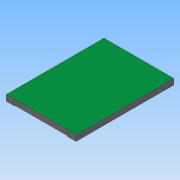
# Autodesk Inventor part: NINA-W102 Body
Saved by Autodesk Inventor 2016 (Build 200138000, 138)
## iProperties
Created: 2019-08-17
Part Number: NINA-W102 Body
Material: Generic
Document SubType Name: Modeling
Designer: Orest
Mass: 0.113046 g
Surface Area: 3.2498 cm^2
Volume: 0.113046 cm^3
Density: 1 g/cm^3
Appearance: Default
Author: Orest
Autodesk Inventor part; units mm, degrees
ref_plane "YZ Plane" through (0, 0, 0) normal (1, 0, 0) x (0, 1, 0)
ref_plane "XZ Plane" through (0, 0, 0) normal (0, 1, 0) x (-1, 0, 0)
ref_plane "XY Plane" through (0, 0, 0) normal (0, 0, 1) x (1, 0, 0)
sketch "Sketch10" plane through (0, 0, 0) normal (0, 1, 0) x (-1, 0, 0)
  line L0 (7, -5) -> (-7, -5)
  line L1 (-7, -5) -> (-7, 5)
  line L2 (-7, 5) -> (7, 5)
  line L3 (6.9, -3.35) -> (6.9, 3.35)
  line L4 (7, 5) -> (7, 3.9745)
  line L5 (7, -3.9745) -> (7, -5)
  line L6 (-7, 0) -> (6.9, 0) construction
  arc A0 (6.9, -3.35) -> (7, -3.9745) centre (8.9, -3.35) ccw
  arc A1 (7, 3.9745) -> (6.9, 3.35) centre (8.9, 3.35) ccw
  point P0 (0, 0)
  point P1 (0, -5)
  dimension "d7" = 14
  dimension "d8" = 10
  dimension "d9" = 0.1
  dimension "d11" = 1.65
  dimension "d12" = 2
  constraints: 14 end point, 4 point on circle, 3 midpoint, 3 parallel, 2 centre point, 2 horizontal, 1 collinear, 1 horizontal alignment, 1 perpendicular, 1 tangent, 1 vertical, 1 vertical alignment, 1 other
  measures "d7" distance of L1.end L2.end
  measures "d8" distance of L0.end L1.end
  measures "d9" distance between parallel lines of L3 L4
  measures "d11" distance from line of L3.start L0
  measures "d12" radius of A0
extrude "Extrusion4" add sketch "Sketch10" along normal blind 0.8
sketch "Sketch11" plane through (0, 0, 0) normal (0, -1, 0) x (1, 0, 0)
  line L0 (-6.45, 4.7) -> (-5.75, 4.7)
  line L1 (-5.75, 4.7) -> (-5.75, 3.55)
  line L2 (-5.75, 3.55) -> (-6.45, 3.55)
  line L3 (-6.45, 3.55) -> (-6.45, 4.7)
  line L4 (-7, -5) -> (7, -5) construction
  line L5 (7, -5) -> (7, 5) construction
  line L6 (7, 5) -> (-7, 5) construction
  line L7 (-7, 5) -> (-7, 3.9745) construction
  arc A0 (-6.9, 3.35) -> (-7, 3.9745) centre (-8.9, 3.35) ccw construction
  line L8 (-6.9, 3.35) -> (-6.9, -3.35) construction
  arc A1 (-7, -3.9745) -> (-6.9, -3.35) centre (-8.9, -3.35) ccw construction
  line L9 (-7, -3.9745) -> (-7, -5) construction
  line L10 (-5.45, 4.7) -> (-4.75, 4.7)
  line L11 (-4.75, 4.7) -> (-4.75, 3.55)
  line L12 (-4.75, 3.55) -> (-5.45, 3.55)
  line L13 (-5.45, 3.55) -> (-5.45, 4.7)
  line L14 (-4.45, 4.7) -> (-3.75, 4.7)
  line L15 (-3.75, 4.7) -> (-3.75, 3.55)
  line L16 (-3.75, 3.55) -> (-4.45, 3.55)
  line L17 (-4.45, 3.55) -> (-4.45, 4.7)
  line L18 (-3.45, 4.7) -> (-2.75, 4.7)
  line L19 (-2.75, 4.7) -> (-2.75, 3.55)
  line L20 (-2.75, 3.55) -> (-3.45, 3.55)
  line L21 (-3.45, 3.55) -> (-3.45, 4.7)
  line L22 (-2.45, 4.7) -> (-1.75, 4.7)
  line L23 (-1.75, 4.7) -> (-1.75, 3.55)
  line L24 (-1.75, 3.55) -> (-2.45, 3.55)
  line L25 (-2.45, 3.55) -> (-2.45, 4.7)
  line L26 (-1.45, 4.7) -> (-0.75, 4.7)
  line L27 (-0.75, 4.7) -> (-0.75, 3.55)
  line L28 (-0.75, 3.55) -> (-1.45, 3.55)
  line L29 (-1.45, 3.55) -> (-1.45, 4.7)
  line L30 (-0.45, 4.7) -> (0.25, 4.7)
  line L31 (0.25, 4.7) -> (0.25, 3.55)
  line L32 (0.25, 3.55) -> (-0.45, 3.55)
  line L33 (-0.45, 3.55) -> (-0.45, 4.7)
  line L34 (0.55, 4.7) -> (1.25, 4.7)
  line L35 (1.25, 4.7) -> (1.25, 3.55)
  line L36 (1.25, 3.55) -> (0.55, 3.55)
  line L37 (0.55, 3.55) -> (0.55, 4.7)
  line L38 (1.55, 4.7) -> (2.25, 4.7)
  line L39 (2.25, 4.7) -> (2.25, 3.55)
  line L40 (2.25, 3.55) -> (1.55, 3.55)
  line L41 (1.55, 3.55) -> (1.55, 4.7)
  line L42 (2.55, 4.7) -> (3.25, 4.7)
  line L43 (3.25, 4.7) -> (3.25, 3.55)
  line L44 (3.25, 3.55) -> (2.55, 3.55)
  line L45 (2.55, 3.55) -> (2.55, 4.7)
  line L46 (-6.6, 2.35) -> (-5.45, 2.35)
  line L47 (-5.45, 2.35) -> (-5.45, 1.65)
  line L48 (-5.45, 1.65) -> (-6.6, 1.65)
  line L49 (-6.6, 1.65) -> (-6.6, 2.35)
  line L50 (-5.45, 1.35) -> (-5.45, 0.65)
  line L51 (-6.6, 1.35) -> (-5.45, 1.35)
  line L52 (-5.45, 0.65) -> (-6.6, 0.65)
  line L53 (-6.6, 0.65) -> (-6.6, 1.35)
  line L54 (-5.45, 0.35) -> (-5.45, -0.35)
  line L55 (-6.6, 0.35) -> (-5.45, 0.35)
  line L56 (-5.45, -0.35) -> (-6.6, -0.35)
  line L57 (-6.6, -0.35) -> (-6.6, 0.35)
  line L58 (-5.45, -0.65) -> (-5.45, -1.35)
  line L59 (-6.6, -0.65) -> (-5.45, -0.65)
  line L60 (-5.45, -1.35) -> (-6.6, -1.35)
  line L61 (-6.6, -1.35) -> (-6.6, -0.65)
  line L62 (-5.45, -1.65) -> (-5.45, -2.35)
  line L63 (-6.6, -1.65) -> (-5.45, -1.65)
  line L64 (-5.45, -2.35) -> (-6.6, -2.35)
  line L65 (-6.6, -2.35) -> (-6.6, -1.65)
  line L66 (-6.9, 0) -> (7, 0) construction
  line L67 (-5, 3.1) -> (-4.3, 3.1)
  line L68 (-4.3, 3.1) -> (-4.3, 2.4)
  line L69 (-4.3, 2.4) -> (-5, 2.4)
  line L70 (-5, 2.4) -> (-5, 3.1)
  line L71 (-4.3, 2) -> (-4.3, 1.3)
  line L72 (-5, 1.3) -> (-5, 2)
  line L73 (-5, 2) -> (-4.3, 2)
  line L74 (-4.3, 1.3) -> (-5, 1.3)
  line L75 (-4.3, 0.9) -> (-4.3, 0.2)
  line L76 (-5, 0.2) -> (-5, 0.9)
  line L77 (-5, 0.9) -> (-4.3, 0.9)
  line L78 (-4.3, 0.2) -> (-5, 0.2)
  line L79 (-4.3, -0.2) -> (-4.3, -0.9)
  line L80 (-5, -0.9) -> (-5, -0.2)
  line L81 (-5, -0.2) -> (-4.3, -0.2)
  line L82 (-4.3, -0.9) -> (-5, -0.9)
  line L83 (-4.3, -1.3) -> (-4.3, -2)
  line L84 (-5, -2) -> (-5, -1.3)
  line L85 (-5, -1.3) -> (-4.3, -1.3)
  line L86 (-4.3, -2) -> (-5, -2)
  line L87 (-4.3, -2.4) -> (-4.3, -3.1)
  line L88 (-5, -3.1) -> (-5, -2.4)
  line L89 (-5, -2.4) -> (-4.3, -2.4)
  line L90 (-4.3, -3.1) -> (-5, -3.1)
  line L91 (-3.67, 0.92) -> (-2.97, 0.92)
  line L92 (-2.97, 0.92) -> (-2.97, 0.22)
  line L93 (-2.97, 0.22) -> (-3.67, 0.22)
  line L94 (-3.67, 0.22) -> (-3.67, 0.92)
  line L95 (-2.52, 0.22) -> (-2.52, 0.92)
  line L96 (-2.52, 0.92) -> (-1.82, 0.92)
  line L97 (-1.82, 0.92) -> (-1.82, 0.22)
  line L98 (-1.82, 0.22) -> (-2.52, 0.22)
  line L99 (-1.37, 0.22) -> (-1.37, 0.92)
  line L100 (-1.37, 0.92) -> (-0.67, 0.92)
  line L101 (-0.67, 0.92) -> (-0.67, 0.22)
  line L102 (-0.67, 0.22) -> (-1.37, 0.22)
  line L103 (-0.22, 0.22) -> (-0.22, 0.92)
  line L104 (-0.22, 0.92) -> (0.48, 0.92)
  line L105 (0.48, 0.92) -> (0.48, 0.22)
  line L106 (0.48, 0.22) -> (-0.22, 0.22)
  line L107 (-3.67, -0.93) -> (-3.67, -0.23)
  line L108 (-3.67, -0.23) -> (-2.97, -0.23)
  line L109 (-2.97, -0.23) -> (-2.97, -0.93)
  line L110 (-2.97, -0.93) -> (-3.67, -0.93)
  line L111 (-2.52, -0.93) -> (-2.52, -0.23)
  line L112 (-2.52, -0.23) -> (-1.82, -0.23)
  line L113 (-1.82, -0.23) -> (-1.82, -0.93)
  line L114 (-1.82, -0.93) -> (-2.52, -0.93)
  line L115 (-1.37, -0.93) -> (-1.37, -0.23)
  line L116 (-1.37, -0.23) -> (-0.67, -0.23)
  line L117 (-0.67, -0.23) -> (-0.67, -0.93)
  line L118 (-0.67, -0.93) -> (-1.37, -0.93)
  line L119 (-0.22, -0.93) -> (-0.22, -0.23)
  line L120 (-0.22, -0.23) -> (0.48, -0.23)
  line L121 (0.48, -0.23) -> (0.48, -0.93)
  line L122 (0.48, -0.93) -> (-0.22, -0.93)
  line L123 (-2.52, 1.37) -> (-2.52, 2.07)
  line L124 (-2.52, 2.07) -> (-1.82, 2.07)
  line L125 (-1.82, 2.07) -> (-1.82, 1.37)
  line L126 (-1.82, 1.37) -> (-2.52, 1.37)
  line L127 (-0.22, 1.37) -> (-0.22, 2.07)
  line L128 (-0.22, 2.07) -> (0.48, 2.07)
  line L129 (0.48, 2.07) -> (0.48, 1.37)
  line L130 (0.48, 1.37) -> (-0.22, 1.37)
  line L131 (-1.82, -2.08) -> (-2.52, -2.08)
  line L132 (-2.52, -2.08) -> (-2.52, -1.38)
  line L133 (-2.52, -1.38) -> (-1.82, -1.38)
  line L134 (-1.82, -1.38) -> (-1.82, -2.08)
  line L135 (0.48, -2.08) -> (-0.22, -2.08)
  line L136 (-0.22, -2.08) -> (-0.22, -1.38)
  line L137 (-0.22, -1.38) -> (0.48, -1.38)
  line L138 (0.48, -1.38) -> (0.48, -2.08)
  line L139 (2.25, 2.35) -> (3.4, 2.35)
  line L140 (3.4, 2.35) -> (3.4, 1.65)
  line L141 (3.4, 1.65) -> (2.25, 1.65)
  line L142 (2.25, 1.65) -> (2.25, 2.35)
  line L143 (2.25, 0.65) -> (2.25, 1.35)
  line L144 (2.25, 1.35) -> (3.4, 1.35)
  line L145 (3.4, 0.65) -> (2.25, 0.65)
  line L146 (3.4, 1.35) -> (3.4, 0.65)
  line L147 (2.25, -0.35) -> (2.25, 0.35)
  line L148 (2.25, 0.35) -> (3.4, 0.35)
  line L149 (3.4, -0.35) -> (2.25, -0.35)
  line L150 (3.4, 0.35) -> (3.4, -0.35)
  line L151 (2.25, -1.35) -> (2.25, -0.65)
  line L152 (2.25, -0.65) -> (3.4, -0.65)
  line L153 (3.4, -1.35) -> (2.25, -1.35)
  line L154 (3.4, -0.65) -> (3.4, -1.35)
  line L155 (2.25, -2.35) -> (2.25, -1.65)
  line L156 (2.25, -1.65) -> (3.4, -1.65)
  line L157 (3.4, -2.35) -> (2.25, -2.35)
  line L158 (3.4, -1.65) -> (3.4, -2.35)
  line L159 (-6.45, -4.7) -> (-5.75, -4.7)
  line L160 (-5.75, -4.7) -> (-5.75, -3.55)
  line L161 (-5.75, -3.55) -> (-6.45, -3.55)
  line L162 (-6.45, -3.55) -> (-6.45, -4.7)
  line L163 (-5.45, -4.7) -> (-4.75, -4.7)
  line L164 (-4.75, -4.7) -> (-4.75, -3.55)
  line L165 (-4.75, -3.55) -> (-5.45, -3.55)
  line L166 (-5.45, -3.55) -> (-5.45, -4.7)
  line L167 (-4.45, -4.7) -> (-3.75, -4.7)
  line L168 (-3.75, -4.7) -> (-3.75, -3.55)
  line L169 (-3.75, -3.55) -> (-4.45, -3.55)
  line L170 (-4.45, -3.55) -> (-4.45, -4.7)
  line L171 (-3.45, -4.7) -> (-2.75, -4.7)
  line L172 (-2.75, -4.7) -> (-2.75, -3.55)
  line L173 (-2.75, -3.55) -> (-3.45, -3.55)
  line L174 (-3.45, -3.55) -> (-3.45, -4.7)
  line L175 (-2.45, -4.7) -> (-1.75, -4.7)
  line L176 (-1.75, -4.7) -> (-1.75, -3.55)
  line L177 (-1.75, -3.55) -> (-2.45, -3.55)
  line L178 (-2.45, -3.55) -> (-2.45, -4.7)
  line L179 (-1.45, -4.7) -> (-0.75, -4.7)
  line L180 (-0.75, -4.7) -> (-0.75, -3.55)
  line L181 (-0.75, -3.55) -> (-1.45, -3.55)
  line L182 (-1.45, -3.55) -> (-1.45, -4.7)
  line L183 (-0.45, -4.7) -> (0.25, -4.7)
  line L184 (0.25, -4.7) -> (0.25, -3.55)
  line L185 (0.25, -3.55) -> (-0.45, -3.55)
  line L186 (-0.45, -3.55) -> (-0.45, -4.7)
  line L187 (0.55, -4.7) -> (1.25, -4.7)
  line L188 (1.25, -4.7) -> (1.25, -3.55)
  line L189 (1.25, -3.55) -> (0.55, -3.55)
  line L190 (0.55, -3.55) -> (0.55, -4.7)
  line L191 (1.55, -4.7) -> (2.25, -4.7)
  line L192 (2.25, -4.7) -> (2.25, -3.55)
  line L193 (2.25, -3.55) -> (1.55, -3.55)
  line L194 (1.55, -3.55) -> (1.55, -4.7)
  line L195 (2.55, -4.7) -> (3.25, -4.7)
  line L196 (3.25, -4.7) -> (3.25, -3.55)
  line L197 (3.25, -3.55) -> (2.55, -3.55)
  line L198 (2.55, -3.55) -> (2.55, -4.7)
  point P0 (0, 0)
  point P1 (-5.45, 0)
  dimension "d17" = 1
  dimension "d22" = 0.7
  dimension "d23" = 0.45
  dimension "d24" = 1.15
  dimension "d25" = 0.3
  dimension "d28" = 1
  dimension "d33" = 0.3
  dimension "d34" = 0.7
  dimension "d37" = 1.1
  dimension "d42" = 1.6
  dimension "d43" = 1.45
  dimension "d47" = 1.15
  dimension "d50" = 1.15
  dimension "d53" = 1.15
  dimension "d54" = 1.15
  dimension "d56" = 2.63
  dimension "d58" = 2.78
  dimension "d59" = 8.7
  dimension "d62" = 1
  constraints: 386 end point, 40 symmetric about line, 15 equal length, 15 perpendicular, 10 parallel, 7 collinear, 7 horizontal, 4 vertical, 3 midpoint, 1 point on line, 232 other
  measures "d17" distance of L0.start L10.start
  measures "d22" distance between parallel lines of L3 L1
  measures "d23" distance between parallel lines of L3 L8
  measures "d24" distance between parallel lines of L2 L0
  measures "d25" distance between parallel lines of L6 L0
  measures "d28" distance of L46.end L50.start
  measures "d33" distance between parallel lines of L8 L65
  measures "d34" distance of L67.start L67.end
  measures "d37" distance of L68.end L71.end
  measures "d42" distance between parallel lines of L0 L67
  measures "d43" distance between parallel lines of L70 L3
  measures "d47" distance of L94.end L95.end
  measures "d50" distance of L94.end L107.end
  measures "d53" distance between parallel lines of L96 L124
  measures "d54" distance between parallel lines of L114 L131
  measures "d56" distance between parallel lines of L124 L0
  measures "d58" distance between parallel lines of L94 L3
  measures "d59" distance between parallel lines of L142 L3
  measures "d62" distance of L139.start L143.end
extrude "Extrusion5" add sketch "Sketch11" along normal blind 0.05
equation "\"d28\" = d17"
equation "\"d33\" = d25"
equation "\"d50\" = d47"
equation "\"d53\" = d47"
equation "\"d54\" = d47"
equation "\"d62\" = d28"
body "Solid4"
